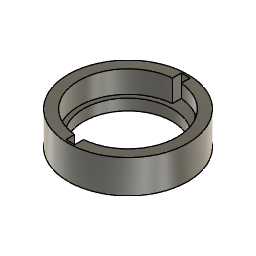
PipeCollar (Autodesk Fusion 360 design; units mm, degrees)
Autodesk Fusion 360 part; units mm, degrees
sketch "Sketch1" plane through (0, 0, 0) normal (0, 0, 1) x (1, 0, 0)
  circle A0 centre (0, 0) radius 27
  dimension "d1" = 54
  constraint coincident A0.centre origin
  measures "d1" diameter of A0
extrude "Extrude1" add sketch "Sketch1" along normal blind 30
sketch "Sketch2" plane through (0, 0, 30) normal (0, 0, 1) x (-1, 0, 0)
  circle A0 centre (0, 0) radius 27
  circle A1 centre (0, 0) radius 20.1
  dimension "d4" = 40.2
  constraint coincident A0.centre A1.centre
  measures "d4" diameter of A1
extrude "Extrude2" cut sketch "Sketch2" against normal blind 30 contours A1
sketch "Sketch9" plane through (0, 0, 30) normal (0, 0, 1) x (-1, 0, 0)
  circle A0 centre (0, 0) radius 20.1
  circle A1 centre (0, 0) radius 27
  circle A2 centre (0, 0) radius 22.2
  dimension "d50" = 44.4
  constraint coincident A0.centre A1.centre
  measures "d50" diameter of A2
extrude "Extrude8" cut sketch "Sketch9" against normal blind 10 contours A2
sketch "Sketch10" plane through (0, 0, 30) normal (0, 0, 1) x (-1, 0, 0)
  circle A0 centre (0, 0) radius 22.2
  circle A1 centre (0, 0) radius 27
  line L0 (2, 26.1) -> (2, 21.6)
  line L1 (2, 26.1) -> (-2, 26.1)
  line L2 (-2, 26.1) -> (-2, 21.6)
  line L3 (-2, 21.6) -> (2, 21.6)
  dimension "d55" = 4.5
  dimension "d56" = 4.5
  constraint perpendicular L0 L1
  constraint perpendicular L1 L2
  constraint perpendicular L0 L3
  measures "d55" distance of L0.start L0.end
  measures "d56" distance of L1.end L2.end
extrude "Extrude9" cut sketch "Sketch10" against normal blind 10 contours A0 L0 L1 L2
ref_plane "WorkPlane4" through (0, -24.1049, 25) normal (1, 0, 0) x (0, -1, 0)
sketch "Sketch12" plane through (0, -24.0547, 25) normal (1, 0, 0) x (0, 1, 0)
  line L0 (-2.122, -5) -> (3, -5)
  line L1 (-2.122, -5) -> (-2.122, -1)
  line L2 (-2.122, -1) -> (3, -1)
  line L3 (3, -1) -> (3, -5)
  dimension "d63" = 4
  dimension "d64" = 5.122
  constraint horizontal L0
  constraint perpendicular L0 L1
  constraint perpendicular L1 L2
  constraint perpendicular L0 L3
  measures "d63" distance of L0.start L1.end
  measures "d64" distance of L0.start L0.end
revolve "Revolve1" cut sketch "Sketch12" angle 30 about axis through (0, 0, 0) along (0, 0, -1)
pattern_circular "C-Pattern1" count 2 over 360 about axis through (0, 0, 1.75) along (0, 0, 1) of "Extrude9", "Revolve1"
sketch "Sketch13" plane through (0, 0, 0) normal (0, 0, -1) x (1, 0, 0)
  circle A0 centre (0, 0) radius 20.1
  circle A1 centre (0, 0) radius 27
  circle A2 centre (0, 0) radius 27
  constraint coincident A0.centre A1.centre
extrude "Extrude10" cut sketch "Sketch13" against normal blind 15
equation "d1 = OuterrDiam"
equation "d4 = LowerInnerDiam + PipeTol"
equation "PipeTol = 0.2 mm"
equation "LowerInnerDiam = 40 mm"
equation "OuterrDiam = 54 mm"
equation "AnchorDiam = 3.6 mm"
equation "AnchorFillet = 3 mm"
equation "d50 = UpperInnerDiam + PipeTol"
equation "UpperInnerDiam = 44.2 mm"
